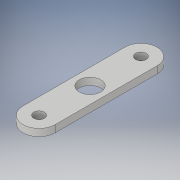
# Autodesk Inventor part: HarmonicDrive-WaveGenerator
Saved by Autodesk Inventor 2018.3 (Build 223284000, 284)
## iProperties
Created: 2018-06-23
Part Number: HarmonicDrive-WaveGenerator
Material: Generisch
Document SubType Name: Modeling
Designer: JochenAlt
Density: 1 g/cm^3
Appearance: Vorgabe
Author: JochenAlt
Autodesk Inventor part; units mm, degrees
ref_plane "YZ Plane" through (0, 0, 0) normal (1, 0, 0) x (0, 1, 0)
ref_plane "XZ Plane" through (0, 0, 0) normal (0, 1, 0) x (-1, 0, 0)
ref_plane "XY Plane" through (0, 0, 0) normal (0, 0, 1) x (1, 0, 0)
sketch "Skizze1" plane through (0, 0, 0) normal (0, 0, 1) x (1, 0, 0)
  line L0 (0, -14.25) -> (0, 14.25) construction
  line L1 (4.5, -14.25) -> (4.5, 14.25)
  line L2 (-4.5, 14.25) -> (-4.5, -14.25)
  arc A0 (-4.5, -14.25) -> (4.5, -14.25) centre (0, -14.25) ccw
  arc A1 (4.5, 14.25) -> (-4.5, 14.25) centre (0, 14.25) ccw
  line L3 (0, 28.35) -> (0, -28.35) construction
  line L4 (-8.4, 0) -> (8.4, 0) construction
  circle A2 centre (0, 14.25) radius 1.5
  circle A3 centre (0, -14.25) radius 1.5
  circle A4 centre (0, 0) radius 3
  circle A5 centre (0, 14.25) radius 6 construction
  circle A6 centre (0, -14.25) radius 6 construction
  line L5 (0, 20.25) -> (0, -20.25) construction
  dimension "d4" = 12
  dimension "d1" = 3
  dimension "d2" = 3
  dimension "d3" = 6
  dimension "d5" = 40.5
  constraints: 10 end point, 5 centre point, 5 coincident, 4 point on circle, 4 tangent, 2 point on line, 2 vertical alignment, 1 equal radius, 1 midpoint, 1 parallel, 1 vertical, 4 other
  measures "d1" diameter of A2
  measures "d2" radial gap between concentric circles of A1 A2
  measures "d3" diameter of A4
  measures "d5" distance of L5.start L5.end
extrude "Extrusion1" add sketch "Skizze1" along normal blind 2
